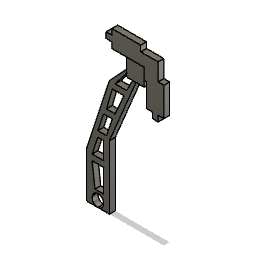
arma_1_(version_minecraft)_v2 (Autodesk Fusion 360 design; units mm, degrees)
Autodesk Fusion 360 part; units mm, degrees
sketch "Boceto1" plane through (0, 0, 0) normal (0, 0, 1) x (1, 0, 0)
sketch "Boceto2" plane through (0, 0, 0) normal (0, 0, 1) x (1, 0, 0)
  line L0 (0, 0) -> (0, 77.2995)
  line L1 (0, 77.2995) -> (40, 200)
  line L2 (40, 200) -> (77.2455, 240)
  line L3 (77.2455, 240) -> (94.1667, 240)
  line L4 (94.1667, 240) -> (40, 110)
  line L5 (40, 110) -> (40, 0)
  line L6 (40, 0) -> (0, 0)
  line L7 (73, 230) -> (85, 230)
  line L8 (85, 230) -> (70, 200)
  line L9 (70, 200) -> (50, 200)
  line L10 (50, 200) -> (73, 230)
  line L11 (45, 190) -> (65, 190)
  line L12 (65, 190) -> (50, 155)
  line L13 (50, 155) -> (35, 155)
  line L14 (35, 155) -> (45, 190)
  line L15 (30, 145) -> (45, 145)
  line L16 (45, 145) -> (35, 115)
  line L17 (35, 115) -> (20, 115)
  line L18 (20, 115) -> (30, 145)
  line L19 (20, 105) -> (30, 105)
  line L20 (30, 105) -> (30, 75)
  line L21 (30, 75) -> (10, 75)
  line L22 (10, 75) -> (20, 105)
  line L23 (10, 65) -> (30, 65)
  line L24 (30, 65) -> (30, 25)
  line L25 (30, 25) -> (15, 25)
  line L26 (15, 25) -> (10, 65)
  constraint coincident L0.start L6.end
  constraint vertical L0
  constraint perpendicular L0 L3
  constraint vertical L5
  constraint perpendicular L0 L6
  constraint horizontal L7
  constraint parallel L7 L9
  constraint horizontal L11
  constraint parallel L11 L13
  constraint horizontal L15
  constraint parallel L15 L17
  constraint parallel L16 L18
  constraint horizontal L19
  constraint perpendicular L19 L20
  constraint perpendicular L20 L21
  constraint horizontal L23
  constraint perpendicular L23 L24
  constraint perpendicular L24 L25
extrude "Extruir1" add sketch "Boceto2" along normal blind 10 makes body 1
cylinder "CilindroPrimitivo1" add diameter 47.743 height 10 placed x (1, 0, 0) y (0, 1, 0) z (0, 0, 1) at (20, 10, 10) separate body makes body 2
copy_body "CopiarPegarCuerpos1" bodies 2 makes body 3
move_body "Desplazar1" bodies 3 to x (1, 0, 0) y (0, 1, 0) z (0, 0, 1) at (0, 0, -20)
hole "Agujero1" at (20.2379, 10.8287, -10) direction (0, 0, 1) diameter 20 depth 20 tip angle 118 bodies 1 2 3
hole "Agujero2" at (20, 10, 20) direction (0, 0, -1) diameter 20 depth 20 tip angle 118 bodies 1 2 3
sketch "Boceto4" plane through (0, 0, 0) normal (0, 0, 1) x (1, 0, 0)
sketch "Boceto5" plane through (0, 0, 10) normal (0, 0, 1) x (1, 0, 0)
  arc A0 (10.5162, 13.1713) -> (20, 0) centre (20, 10) ccw
  arc A1 (29.7218, 7.6575) -> (10.5162, 13.1713) centre (20.2379, 10.8287) ccw
  arc A2 (20, 0) -> (29.7218, 7.6575) centre (20, 10) ccw
  line L0 (20, 0) -> (40, 0)
  line L1 (40, 0) -> (40, 110)
  line L2 (40, 110) -> (94.1667, 240)
  line L3 (94.1667, 240) -> (77.2455, 240)
  line L4 (77.2455, 240) -> (40, 200)
  line L5 (40, 200) -> (0, 77.2995)
  line L6 (0, 77.2995) -> (0, 0)
  line L7 (0, 0) -> (20, 0)
  line L8 (70, 200) -> (50, 200)
  line L9 (50, 200) -> (73, 230)
  line L10 (73, 230) -> (85, 230)
  line L11 (85, 230) -> (70, 200)
  line L12 (50, 155) -> (35, 155)
  line L13 (35, 155) -> (45, 190)
  line L14 (45, 190) -> (65, 190)
  line L15 (65, 190) -> (50, 155)
  line L16 (35, 115) -> (20, 115)
  line L17 (20, 115) -> (30, 145)
  line L18 (30, 145) -> (45, 145)
  line L19 (45, 145) -> (35, 115)
  line L20 (30, 75) -> (10, 75)
  line L21 (10, 75) -> (20, 105)
  line L22 (20, 105) -> (30, 105)
  line L23 (30, 105) -> (30, 75)
  line L24 (30, 25) -> (15, 25)
  line L25 (15, 25) -> (10, 65)
  line L26 (10, 65) -> (30, 65)
  line L27 (30, 65) -> (30, 25)
  line L28 (50, 340) -> (50, 330)
  line L29 (50, 330) -> (60, 330)
  line L30 (60, 330) -> (60, 320)
  line L31 (60, 320) -> (100, 320)
  line L32 (100, 320) -> (100, 310)
  line L33 (100, 310) -> (110, 310)
  line L34 (110, 310) -> (110, 300)
  line L35 (110, 300) -> (120, 300)
  line L36 (120, 300) -> (120, 260)
  line L37 (120, 260) -> (130, 260)
  line L38 (130, 260) -> (130, 250)
  line L39 (130, 250) -> (140, 250)
  line L40 (140, 250) -> (140, 260)
  line L41 (140, 260) -> (150, 260)
  line L42 (150, 260) -> (150, 310)
  line L43 (150, 310) -> (140, 310)
  line L44 (140, 310) -> (140, 340)
  line L45 (140, 340) -> (110, 340)
  line L46 (110, 340) -> (110, 350)
  line L47 (110, 350) -> (60, 350)
  line L48 (60, 350) -> (60, 340)
  line L49 (60, 340) -> (50, 340)
  constraint vertical L28
  constraint perpendicular L28 L29
  constraint perpendicular L29 L30
  constraint perpendicular L30 L31
  constraint perpendicular L29 L32
  constraint perpendicular L32 L33
  constraint perpendicular L33 L34
  constraint perpendicular L34 L35
  constraint perpendicular L35 L36
  constraint perpendicular L36 L37
  constraint perpendicular L37 L38
  constraint perpendicular L38 L39
  constraint perpendicular L39 L40
  constraint perpendicular L40 L41
  constraint perpendicular L41 L42
  constraint perpendicular L42 L43
  constraint perpendicular L43 L44
  constraint perpendicular L44 L45
  constraint perpendicular L43 L46
  constraint perpendicular L46 L47
  constraint perpendicular L47 L48
  constraint perpendicular L28 L49
extrude "Extruir2" add sketch "Boceto5" along normal blind 10 separate body contours L28 L29 L30 L31 L32 L33 L34 L35 L36 L37 L38 L39 L40 L41 L42 L43 L44 L45 L46 L47 L48 L49 makes body 4
move_body "Desplazar2" bodies 4 to x (1, 0, 0) y (0, 1, 0) z (0, 0, 1) at (-20.4494, -47.9195, 22.1569)
move_body "Desplazar3" bodies 4 to x (1, 0, 0) y (0, 1, 0) z (0, 0, 1) at (4.6161, -12.0805, -32.1569)
move_body "Desplazar4" bodies 4 to x (1, 0, 0) y (0, 1, 0) z (0, 0, 1) at (0, -10, 0)
box "CajaPrimitiva1" add length 30 width 30 height 10 placed x (0, -1, 0) y (-1, 0, 0) z (0, 0, -1) at (100, 250, 0) separate body makes body 5
box "CajaPrimitiva2" cut length 30 width 30 height 10 placed x (0, -1, 0) y (1, 0, 0) z (0, 0, 1) at (70, 250, 0) bodies 1 4
move_body "Desplazar6" bodies 5 to x (1, 0, 0) y (0, 1, 0) z (0, 0, 1) at (0, 0, 10)
delete_body "QuitarCuerpo1" bodies 2
delete_body "QuitarCuerpo2" bodies 3
scale "Escala1" factor 0.9 about (40, 110, 0) bodies 4 5 1
scale "Escala2" factor 0.8 about (40, 110, 0) bodies 5 4 1
